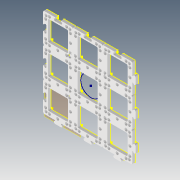
# Autodesk Inventor part: 30_XYTabel_Aliexpress_basplateadapter
Saved by Autodesk Inventor 2022 (Build 260153000, 153)
## iProperties
Created: 2021-11-18
Part Number: 30_XYTabel_Aliexpress_basplateadapter
Material: Generic
Document SubType Name: Modeling
Designer: diederichbenedict
Density: 1 g/cm^3
Appearance: Default
Author: diederichbenedict
Autodesk Inventor part; units mm, degrees
(part 1 of 2)
ref_plane "YZ Plane" through (0, 0, 0) normal (1, 0, 0) x (0, 1, 0)
ref_plane "XZ Plane" through (0, 0, 0) normal (0, 1, 0) x (-1, 0, 0)
ref_plane "XY Plane" through (0, 0, 0) normal (0, 0, 1) x (1, 0, 0)
ref_plane "Work Plane2" through (-50, -50, 0) normal (0, 0, 1) x (1, 0, 0)
sketch "Sketch3" plane through (-50, -50, 0) normal (0, 0, 1) x (1, 0, 0)
  circle A0 centre (5.794757, 15.405243) radius 2.5
  circle A1 centre (-15.605243, -5.794757) radius 2.5
  line L0 (-20.085611, 39.076178) -> (-20.085611, 40.205243)
  line L1 (-20.085611, 40.205243) -> (-38.205243, 40.205243)
  arc A2 (-38.205243, 40.205243) -> (-40.205243, 38.205243) centre (-38.205243, 38.205243) ccw
  line L2 (-40.205243, 20.295345) -> (-40.205243, 38.205243)
  line L3 (-40.205243, 20.295345) -> (-39.078298, 20.295345)
  arc A3 (-39.078298, 20.295345) -> (-38.67683, 20.623155) centre (-39.078298, 20.705088) ccw
  arc A4 (-34.539143, 20.205243) -> (-38.67683, 20.623155) centre (-36.629091, 20.205243) ccw
  line L4 (-34.539143, 20.205243) -> (-34.539143, 10.406652)
  arc A5 (-38.646985, 9.864261) -> (-34.539143, 10.406652) centre (-36.602278, 10.205243) ccw
  line L5 (-38.646985, 9.864261) -> (-38.677461, 9.984929)
  arc A6 (-38.677461, 9.984929) -> (-39.076178, 10.324875) centre (-39.082965, 9.913117) ccw
  line L6 (-39.076178, 10.324875) -> (-40.205243, 10.324875)
  line L7 (-40.205243, -7.794757) -> (-40.205243, 10.324875)
  arc A7 (-40.205243, -7.794757) -> (-38.205243, -9.794757) centre (-38.205243, -7.794757) ccw
  line L8 (-38.205243, -9.794757) -> (-20.205243, -9.794757)
  line L9 (-20.205243, -9.794757) -> (-20.205243, -10.845267)
  arc A8 (-20.605243, -11.335165) -> (-20.205243, -10.845267) centre (-20.705243, -10.845267) ccw
  arc A9 (-20.605243, -11.335165) -> (-20.205243, -15.294757) centre (-20.205243, -13.294757) ccw
  line L10 (-20.205243, -15.294757) -> (-10.205243, -15.294757)
  arc A10 (-10.205243, -15.294757) -> (-9.805243, -11.335165) centre (-10.205243, -13.294757) ccw
  arc A11 (-10.205243, -10.845267) -> (-9.805243, -11.335165) centre (-9.705243, -10.845267) ccw
  line L11 (-10.205243, -10.845267) -> (-10.205243, -9.794757)
  line L12 (-10.205243, -9.794757) -> (7.794757, -9.794757)
  arc A12 (7.794757, -9.794757) -> (9.794757, -7.794757) centre (7.794757, -7.794757) ccw
  line L13 (9.794757, 10.205243) -> (9.794757, -7.794757)
  line L14 (9.794757, 10.205243) -> (10.845267, 10.205243)
  arc A13 (11.335165, 9.805243) -> (10.845267, 10.205243) centre (10.845267, 9.705243) ccw
  arc A14 (11.335165, 9.805243) -> (15.294757, 10.205243) centre (13.294757, 10.205243) ccw
  line L15 (15.294757, 10.205243) -> (15.294757, 20.205243)
  arc A15 (15.294757, 20.205243) -> (11.335165, 20.605243) centre (13.294757, 20.205243) ccw
  arc A16 (10.845267, 20.205243) -> (11.335165, 20.605243) centre (10.845267, 20.705243) ccw
  line L16 (10.845267, 20.205243) -> (9.794757, 20.205243)
  line L17 (9.794757, 38.205243) -> (9.794757, 20.205243)
  arc A17 (9.794757, 38.205243) -> (7.794757, 40.205243) centre (7.794757, 38.205243) ccw
  line L18 (7.794757, 40.205243) -> (-10.115141, 40.205243)
  line L19 (-10.115141, 40.205243) -> (-10.115141, 39.078298)
  arc A18 (-10.115141, 39.078298) -> (-9.787332, 38.67683) centre (-9.705399, 39.078298) ccw
  arc A19 (-10.205243, 34.539143) -> (-9.787332, 38.67683) centre (-10.205243, 36.629091) ccw
  line L20 (-10.205243, 34.539143) -> (-20.003834, 34.539143)
  arc A20 (-20.546226, 38.646985) -> (-20.003834, 34.539143) centre (-20.205243, 36.602278) ccw
  line L21 (-20.546226, 38.646985) -> (-20.425557, 38.677461)
  arc A21 (-20.425557, 38.677461) -> (-20.085611, 39.076178) centre (-20.497369, 39.082965) ccw
  line L22 (-0.205243, 32.205243) -> (-30.205243, 32.205243)
  arc A22 (1.794757, 30.205243) -> (-0.205243, 32.205243) centre (-0.205243, 30.205243) ccw
  line L23 (1.794757, 30.205243) -> (1.794757, 0.205243)
  arc A23 (-0.205243, -1.794757) -> (1.794757, 0.205243) centre (-0.205243, 0.205243) ccw
  line L24 (-0.205243, -1.794757) -> (-30.205243, -1.794757)
  arc A24 (-32.205243, 0.205243) -> (-30.205243, -1.794757) centre (-30.205243, 0.205243) ccw
  line L25 (-32.205243, 0.205243) -> (-32.205243, 30.205243)
  arc A25 (-30.205243, 32.205243) -> (-32.205243, 30.205243) centre (-30.205243, 30.205243) ccw
  circle A26 centre (-35.205243, 35.205243) radius 2.425
  circle A27 centre (-29.705243, 36.005243) radius 2.65 construction
  circle A28 centre (-36.005243, 29.705243) radius 2.65 construction
  circle A29 centre (-35.205243, -4.794757) radius 2.425
  circle A30 centre (-29.705243, -5.594757) radius 2.65 construction
  circle A31 centre (-36.005243, 0.705243) radius 2.65 construction
  circle A32 centre (4.794757, 35.205243) radius 2.425
  circle A33 centre (-0.705243, 36.005243) radius 2.65 construction
  circle A34 centre (5.594757, 29.705243) radius 2.65 construction
  circle A35 centre (5.594757, 0.705243) radius 2.65 construction
  circle A36 centre (-0.705243, -5.594757) radius 2.65 construction
  circle A37 centre (4.794757, -4.794757) radius 2.425
  circle A38 centre (-0.705243, -5.594757) radius 2.6
  circle A39 centre (-29.705243, -5.594757) radius 2.6
  circle A40 centre (-36.005243, 0.705243) radius 2.6
  circle A41 centre (-36.005243, 29.705243) radius 2.6
  circle A42 centre (-29.705243, 36.005243) radius 2.6
  circle A43 centre (-0.705243, 36.005243) radius 2.6
  circle A44 centre (5.594757, 29.705243) radius 2.6
  circle A45 centre (5.594757, 0.705243) radius 2.6
  point P0 (50, 50)
  dimension "d23" = 0.05
  dimension "d24" = 0.05
  dimension "d25" = 0.05
  dimension "d26" = 0.05
  dimension "d27" = 0.05
  dimension "d28" = 0.05
  dimension "d29" = 0.05
  dimension "d30" = 0.05
  constraints: 8 centre point
  measures "d23" radial gap between concentric circles of A36 A38
  measures "d24" radial gap between concentric circles of A30 A39
  measures "d25" radial gap between concentric circles of A31 A40
  measures "d26" radial gap between concentric circles of A28 A41
  measures "d27" radial gap between concentric circles of A27 A42
  measures "d28" radial gap between concentric circles of A33 A43
  measures "d29" radial gap between concentric circles of A34 A44
  measures "d30" radial gap between concentric circles of A35 A45
extrude "Extrusion2" add sketch "Sketch3" along normal blind 5
pattern_linear "Rectangular Pattern1" count 3 spacing 50 along (1, 0, 0) count 3 spacing 50 along (0, 1, 0) of "Extrusion2"
sketch "Sketch4" plane through (-50, -50, 5) normal (0, 0, 1) x (1, 0, 0)
  line L0 (-10.115141, 40.205243) -> (-10.115141, 39.078298)
  arc A0 (-10.115141, 39.078298) -> (-9.787332, 38.67683) centre (-9.705399, 39.078298) ccw
  arc A1 (-10.205243, 34.539143) -> (-9.787332, 38.67683) centre (-10.205243, 36.629091) ccw
  line L1 (-10.205243, 34.539143) -> (-20.003834, 34.539143)
  arc A2 (-21.642091, 38.096455) -> (-20.003834, 34.539143) centre (-20.205243, 36.602278) ccw
  arc A3 (-21.642091, 38.096455) -> (-20.205243, 34.705243) centre (-20.205243, 36.705243) ccw
  line L2 (-20.205243, 34.705243) -> (-10.205243, 34.705243)
  arc A4 (-10.205243, 34.705243) -> (-9.805243, 38.664835) centre (-10.205243, 36.705243) ccw
  arc A5 (-10.205243, 39.154733) -> (-9.805243, 38.664835) centre (-9.705243, 39.154733) ccw
  line L3 (-10.205243, 39.154733) -> (-10.205243, 40.205243)
  line L4 (-10.205243, 40.205243) -> (-10.115141, 40.205243)
  arc A6 (7.794757, 40.205243) -> (9.794757, 42.205243) centre (7.794757, 42.205243) ccw
  arc A7 (9.794757, 42.205243) -> (11.794757, 40.205243) centre (11.794757, 42.205243) ccw
  arc A8 (11.794757, 40.205243) -> (9.794757, 38.205243) centre (11.794757, 38.205243) ccw
  arc A9 (9.794757, 38.205243) -> (7.794757, 40.205243) centre (7.794757, 38.205243) ccw
  line L5 (9.794757, 20.295345) -> (10.921702, 20.295345)
  arc A10 (10.921702, 20.295345) -> (11.32317, 20.623155) centre (10.921702, 20.705088) ccw
  arc A11 (15.460857, 20.205243) -> (11.32317, 20.623155) centre (13.370909, 20.205243) ccw
  line L6 (15.460857, 20.205243) -> (15.460857, 10.406652)
  arc A12 (11.903545, 8.768396) -> (15.460857, 10.406652) centre (13.397722, 10.205243) ccw
  arc A13 (11.903545, 8.768396) -> (15.294757, 10.205243) centre (13.294757, 10.205243) ccw
  line L7 (15.294757, 10.205243) -> (15.294757, 20.205243)
  arc A14 (15.294757, 20.205243) -> (11.335165, 20.605243) centre (13.294757, 20.205243) ccw
  arc A15 (10.845267, 20.205243) -> (11.335165, 20.605243) centre (10.845267, 20.705243) ccw
  line L8 (10.845267, 20.205243) -> (9.794757, 20.205243)
  line L9 (9.794757, 20.205243) -> (9.794757, 20.295345)
  line L10 (39.884859, 90.205243) -> (39.884859, 89.078298)
  arc A16 (39.884859, 89.078298) -> (40.212668, 88.67683) centre (40.294601, 89.078298) ccw
  arc A17 (39.794757, 84.539143) -> (40.212668, 88.67683) centre (39.794757, 86.629091) ccw
  line L11 (39.794757, 84.539143) -> (29.996166, 84.539143)
  arc A18 (28.357909, 88.096455) -> (29.996166, 84.539143) centre (29.794757, 86.602278) ccw
  arc A19 (28.357909, 88.096455) -> (29.794757, 84.705243) centre (29.794757, 86.705243) ccw
  line L12 (29.794757, 84.705243) -> (39.794757, 84.705243)
  arc A20 (39.794757, 84.705243) -> (40.194757, 88.664835) centre (39.794757, 86.705243) ccw
  arc A21 (39.794757, 89.154733) -> (40.194757, 88.664835) centre (40.294757, 89.154733) ccw
  line L13 (39.794757, 89.154733) -> (39.794757, 90.205243)
  line L14 (39.794757, 90.205243) -> (39.884859, 90.205243)
  arc A22 (11.903545, 108.768396) -> (15.294757, 110.205243) centre (13.294757, 110.205243) ccw
  line L15 (15.294757, 110.205243) -> (15.294757, 120.205243)
  arc A23 (15.294757, 120.205243) -> (11.335165, 120.605243) centre (13.294757, 120.205243) ccw
  arc A24 (10.845267, 120.205243) -> (11.335165, 120.605243) centre (10.845267, 120.705243) ccw
  line L16 (10.845267, 120.205243) -> (9.794757, 120.205243)
  line L17 (9.794757, 120.205243) -> (9.794757, 120.295345)
  line L18 (9.794757, 120.295345) -> (10.921702, 120.295345)
  arc A25 (10.921702, 120.295345) -> (11.32317, 120.623155) centre (10.921702, 120.705088) ccw
  arc A26 (15.460857, 120.205243) -> (11.32317, 120.623155) centre (13.370909, 120.205243) ccw
  line L19 (15.460857, 120.205243) -> (15.460857, 110.406652)
  arc A27 (11.903545, 108.768396) -> (15.460857, 110.406652) centre (13.397722, 110.205243) ccw
  arc A28 (9.794757, 92.205243) -> (11.794757, 90.205243) centre (11.794757, 92.205243) ccw
  arc A29 (11.794757, 90.205243) -> (9.794757, 88.205243) centre (11.794757, 88.205243) ccw
  arc A30 (9.794757, 88.205243) -> (7.794757, 90.205243) centre (7.794757, 88.205243) ccw
  arc A31 (7.794757, 90.205243) -> (9.794757, 92.205243) centre (7.794757, 92.205243) ccw
  line L20 (51.794757, 130.205243) -> (51.794757, 100.205243)
  arc A32 (49.794757, 98.205243) -> (51.794757, 100.205243) centre (49.794757, 100.205243) ccw
  line L21 (49.794757, 98.205243) -> (19.794757, 98.205243)
  arc A33 (17.794757, 100.205243) -> (19.794757, 98.205243) centre (19.794757, 100.205243) ccw
  line L22 (17.794757, 100.205243) -> (17.794757, 130.205243)
  arc A34 (19.794757, 132.205243) -> (17.794757, 130.205243) centre (19.794757, 130.205243) ccw
  line L23 (19.794757, 132.205243) -> (49.794757, 132.205243)
  arc A35 (51.794757, 130.205243) -> (49.794757, 132.205243) centre (49.794757, 130.205243) ccw
  circle A36 centre (55.594757, 129.705243) radius 2.6
  circle A37 centre (20.294757, 136.005243) radius 2.6
  circle A38 centre (13.994757, 100.705243) radius 2.6
  circle A39 centre (55.794757, 115.405243) radius 2.5
  circle A40 centre (34.394757, 94.205243) radius 2.5
  circle A41 centre (14.794757, 135.205243) radius 2.425
  circle A42 centre (14.794757, 95.205243) radius 2.425
  circle A43 centre (54.794757, 135.205243) radius 2.425
  circle A44 centre (54.794757, 95.205243) radius 2.425
  circle A45 centre (49.294757, 94.405243) radius 2.6
  circle A46 centre (20.294757, 94.405243) radius 2.6
  circle A47 centre (13.994757, 129.705243) radius 2.6
  circle A48 centre (49.294757, 136.005243) radius 2.6
  circle A49 centre (55.594757, 100.705243) radius 2.6
  line L24 (39.884859, 40.205243) -> (39.884859, 39.078298)
  arc A50 (39.884859, 39.078298) -> (40.212668, 38.67683) centre (40.294601, 39.078298) ccw
  arc A51 (39.794757, 34.539143) -> (40.212668, 38.67683) centre (39.794757, 36.629091) ccw
  line L25 (39.794757, 34.539143) -> (29.996166, 34.539143)
  arc A52 (28.357909, 38.096455) -> (29.996166, 34.539143) centre (29.794757, 36.602278) ccw
  arc A53 (28.357909, 38.096455) -> (29.794757, 34.705243) centre (29.794757, 36.705243) ccw
  line L26 (29.794757, 34.705243) -> (39.794757, 34.705243)
  arc A54 (39.794757, 34.705243) -> (40.194757, 38.664835) centre (39.794757, 36.705243) ccw
  arc A55 (39.794757, 39.154733) -> (40.194757, 38.664835) centre (40.294757, 39.154733) ccw
  line L27 (39.794757, 39.154733) -> (39.794757, 40.205243)
  line L28 (39.794757, 40.205243) -> (39.884859, 40.205243)
  circle A56 centre (5.594757, 50.705243) radius 2.6
  circle A57 centre (-0.705243, 86.005243) radius 2.6
  circle A58 centre (-36.005243, 79.705243) radius 2.6
  circle A59 centre (-29.705243, 44.405243) radius 2.6
  circle A60 centre (-0.705243, 44.405243) radius 2.6
  circle A61 centre (4.794757, 45.205243) radius 2.425
  circle A62 centre (4.794757, 85.205243) radius 2.425
  circle A63 centre (-35.205243, 45.205243) radius 2.425
  circle A64 centre (-35.205243, 85.205243) radius 2.425
  circle A65 centre (-15.605243, 44.205243) radius 2.5
  circle A66 centre (5.794757, 65.405243) radius 2.5
  circle A67 centre (-36.005243, 50.705243) radius 2.6
  circle A68 centre (-29.705243, 86.005243) radius 2.6
  circle A69 centre (5.594757, 79.705243) radius 2.6
  line L29 (1.794757, 80.205243) -> (1.794757, 50.205243)
  arc A70 (-0.205243, 48.205243) -> (1.794757, 50.205243) centre (-0.205243, 50.205243) ccw
  line L30 (-0.205243, 48.205243) -> (-30.205243, 48.205243)
  arc A71 (-32.205243, 50.205243) -> (-30.205243, 48.205243) centre (-30.205243, 50.205243) ccw
  line L31 (-32.205243, 50.205243) -> (-32.205243, 80.205243)
  arc A72 (-30.205243, 82.205243) -> (-32.205243, 80.205243) centre (-30.205243, 80.205243) ccw
  line L32 (-30.205243, 82.205243) -> (-0.205243, 82.205243)
  arc A73 (1.794757, 80.205243) -> (-0.205243, 82.205243) centre (-0.205243, 80.205243) ccw
  line L33 (51.794757, 80.205243) -> (51.794757, 50.205243)
  arc A74 (49.794757, 48.205243) -> (51.794757, 50.205243) centre (49.794757, 50.205243) ccw
  line L34 (49.794757, 48.205243) -> (19.794757, 48.205243)
  arc A75 (17.794757, 50.205243) -> (19.794757, 48.205243) centre (19.794757, 50.205243) ccw
  line L35 (17.794757, 50.205243) -> (17.794757, 80.205243)
  arc A76 (19.794757, 82.205243) -> (17.794757, 80.205243) centre (19.794757, 80.205243) ccw
  line L36 (19.794757, 82.205243) -> (49.794757, 82.205243)
  arc A77 (51.794757, 80.205243) -> (49.794757, 82.205243) centre (49.794757, 80.205243) ccw
  circle A78 centre (55.594757, 79.705243) radius 2.6
  circle A79 centre (20.294757, 86.005243) radius 2.6
  circle A80 centre (13.994757, 50.705243) radius 2.6
  circle A81 centre (55.794757, 65.405243) radius 2.5
  circle A82 centre (34.394757, 44.205243) radius 2.5
  circle A83 centre (14.794757, 85.205243) radius 2.425
  circle A84 centre (14.794757, 45.205243) radius 2.425
  circle A85 centre (54.794757, 85.205243) radius 2.425
  circle A86 centre (54.794757, 45.205243) radius 2.425
  circle A87 centre (49.294757, 44.405243) radius 2.6
  circle A88 centre (20.294757, 44.405243) radius 2.6
  circle A89 centre (13.994757, 79.705243) radius 2.6
  circle A90 centre (49.294757, 86.005243) radius 2.6
  circle A91 centre (55.594757, 50.705243) radius 2.6
  arc A92 (11.903545, 58.768396) -> (15.294757, 60.205243) centre (13.294757, 60.205243) ccw
  line L37 (15.294757, 60.205243) -> (15.294757, 70.205243)
  arc A93 (15.294757, 70.205243) -> (11.335165, 70.605243) centre (13.294757, 70.205243) ccw
  arc A94 (10.845267, 70.205243) -> (11.335165, 70.605243) centre (10.845267, 70.705243) ccw
  line L38 (10.845267, 70.205243) -> (9.794757, 70.205243)
  line L39 (9.794757, 70.205243) -> (9.794757, 70.295345)
  line L40 (9.794757, 70.295345) -> (10.921702, 70.295345)
  arc A95 (10.921702, 70.295345) -> (11.32317, 70.623155) centre (10.921702, 70.705088) ccw
  arc A96 (15.460857, 70.205243) -> (11.32317, 70.623155) centre (13.370909, 70.205243) ccw
  line L41 (15.460857, 70.205243) -> (15.460857, 60.406652)
  arc A97 (11.903545, 58.768396) -> (15.460857, 60.406652) centre (13.397722, 60.205243) ccw
  arc A98 (61.903545, 8.768396) -> (65.294757, 10.205243) centre (63.294757, 10.205243) ccw
  line L42 (65.294757, 10.205243) -> (65.294757, 20.205243)
  arc A99 (65.294757, 20.205243) -> (61.335165, 20.605243) centre (63.294757, 20.205243) ccw
  arc A100 (60.845267, 20.205243) -> (61.335165, 20.605243) centre (60.845267, 20.705243) ccw
  line L43 (60.845267, 20.205243) -> (59.794757, 20.205243)
  line L44 (59.794757, 20.205243) -> (59.794757, 20.295345)
  line L45 (59.794757, 20.295345) -> (60.921702, 20.295345)
  arc A101 (60.921702, 20.295345) -> (61.32317, 20.623155) centre (60.921702, 20.705088) ccw
  arc A102 (65.460857, 20.205243) -> (61.32317, 20.623155) centre (63.370909, 20.205243) ccw
  line L46 (65.460857, 20.205243) -> (65.460857, 10.406652)
  arc A103 (61.903545, 8.768396) -> (65.460857, 10.406652) centre (63.397722, 10.205243) ccw
  line L47 (101.794757, 30.205243) -> (101.794757, 0.205243)
  arc A104 (99.794757, -1.794757) -> (101.794757, 0.205243) centre (99.794757, 0.205243) ccw
  line L48 (99.794757, -1.794757) -> (69.794757, -1.794757)
  arc A105 (67.794757, 0.205243) -> (69.794757, -1.794757) centre (69.794757, 0.205243) ccw
  line L49 (67.794757, 0.205243) -> (67.794757, 30.205243)
  arc A106 (69.794757, 32.205243) -> (67.794757, 30.205243) centre (69.794757, 30.205243) ccw
  line L50 (69.794757, 32.205243) -> (99.794757, 32.205243)
  arc A107 (101.794757, 30.205243) -> (99.794757, 32.205243) centre (99.794757, 30.205243) ccw
  circle A108 centre (105.594757, 29.705243) radius 2.6
  circle A109 centre (70.294757, 36.005243) radius 2.6
  circle A110 centre (63.994757, 0.705243) radius 2.6
  circle A111 centre (105.794757, 15.405243) radius 2.5
  circle A112 centre (84.394757, -5.794757) radius 2.5
  circle A113 centre (64.794757, 35.205243) radius 2.425
  circle A114 centre (64.794757, -4.794757) radius 2.425
  circle A115 centre (104.794757, 35.205243) radius 2.425
  circle A116 centre (104.794757, -4.794757) radius 2.425
  circle A117 centre (99.294757, -5.594757) radius 2.6
  circle A118 centre (70.294757, -5.594757) radius 2.6
  circle A119 centre (63.994757, 29.705243) radius 2.6
  circle A120 centre (99.294757, 36.005243) radius 2.6
  circle A121 centre (105.594757, 0.705243) radius 2.6
  line L51 (51.794757, 30.205243) -> (51.794757, 0.205243)
  arc A122 (49.794757, -1.794757) -> (51.794757, 0.205243) centre (49.794757, 0.205243) ccw
  line L52 (49.794757, -1.794757) -> (19.794757, -1.794757)
  arc A123 (17.794757, 0.205243) -> (19.794757, -1.794757) centre (19.794757, 0.205243) ccw
  line L53 (17.794757, 0.205243) -> (17.794757, 30.205243)
  arc A124 (19.794757, 32.205243) -> (17.794757, 30.205243) centre (19.794757, 30.205243) ccw
  line L54 (19.794757, 32.205243) -> (49.794757, 32.205243)
  arc A125 (51.794757, 30.205243) -> (49.794757, 32.205243) centre (49.794757, 30.205243) ccw
  circle A126 centre (55.594757, 29.705243) radius 2.6
  circle A127 centre (20.294757, 36.005243) radius 2.6
  circle A128 centre (13.994757, 0.705243) radius 2.6
  circle A129 centre (55.794757, 15.405243) radius 2.5
  circle A130 centre (34.394757, -5.794757) radius 2.5
  circle A131 centre (14.794757, 35.205243) radius 2.425
  circle A132 centre (14.794757, -4.794757) radius 2.425
  circle A133 centre (54.794757, 35.205243) radius 2.425
  circle A134 centre (54.794757, -4.794757) radius 2.425
  circle A135 centre (49.294757, -5.594757) radius 2.6
  circle A136 centre (20.294757, -5.594757) radius 2.6
  circle A137 centre (13.994757, 29.705243) radius 2.6
  circle A138 centre (49.294757, 36.005243) radius 2.6
  circle A139 centre (55.594757, 0.705243) radius 2.6
  circle A140 centre (105.594757, 50.705243) radius 2.6
  circle A141 centre (99.294757, 86.005243) radius 2.6
  circle A142 centre (63.994757, 79.705243) radius 2.6
  circle A143 centre (70.294757, 44.405243) radius 2.6
  circle A144 centre (99.294757, 44.405243) radius 2.6
  circle A145 centre (104.794757, 45.205243) radius 2.425
  circle A146 centre (104.794757, 85.205243) radius 2.425
  circle A147 centre (64.794757, 45.205243) radius 2.425
  circle A148 centre (64.794757, 85.205243) radius 2.425
  circle A149 centre (84.394757, 44.205243) radius 2.5
  circle A150 centre (105.794757, 65.405243) radius 2.5
  circle A151 centre (63.994757, 50.705243) radius 2.6
  circle A152 centre (70.294757, 86.005243) radius 2.6
  circle A153 centre (105.594757, 79.705243) radius 2.6
  line L55 (101.794757, 80.205243) -> (101.794757, 50.205243)
  arc A154 (99.794757, 48.205243) -> (101.794757, 50.205243) centre (99.794757, 50.205243) ccw
  line L56 (99.794757, 48.205243) -> (69.794757, 48.205243)
  arc A155 (67.794757, 50.205243) -> (69.794757, 48.205243) centre (69.794757, 50.205243) ccw
  line L57 (67.794757, 50.205243) -> (67.794757, 80.205243)
  arc A156 (69.794757, 82.205243) -> (67.794757, 80.205243) centre (69.794757, 80.205243) ccw
  line L58 (69.794757, 82.205243) -> (99.794757, 82.205243)
  arc A157 (101.794757, 80.205243) -> (99.794757, 82.205243) centre (99.794757, 80.205243) ccw
  arc A158 (59.794757, 42.205243) -> (61.794757, 40.205243) centre (61.794757, 42.205243) ccw
  arc A159 (61.794757, 40.205243) -> (59.794757, 38.205243) centre (61.794757, 38.205243) ccw
  arc A160 (59.794757, 38.205243) -> (57.794757, 40.205243) centre (57.794757, 38.205243) ccw
  arc A161 (57.794757, 40.205243) -> (59.794757, 42.205243) centre (57.794757, 42.205243) ccw
  arc A162 (61.903545, 58.768396) -> (65.294757, 60.205243) centre (63.294757, 60.205243) ccw
  line L59 (65.294757, 60.205243) -> (65.294757, 70.205243)
  arc A163 (65.294757, 70.205243) -> (61.335165, 70.605243) centre (63.294757, 70.205243) ccw
  arc A164 (60.845267, 70.205243) -> (61.335165, 70.605243) centre (60.845267, 70.705243) ccw
  line L60 (60.845267, 70.205243) -> (59.794757, 70.205243)
  line L61 (59.794757, 70.205243) -> (59.794757, 70.295345)
  line L62 (59.794757, 70.295345) -> (60.921702, 70.295345)
  arc A165 (60.921702, 70.295345) -> (61.32317, 70.623155) centre (60.921702, 70.705088) ccw
  arc A166 (65.460857, 70.205243) -> (61.32317, 70.623155) centre (63.370909, 70.205243) ccw
  line L63 (65.460857, 70.205243) -> (65.460857, 60.406652)
  arc A167 (61.903545, 58.768396) -> (65.460857, 60.406652) centre (63.397722, 60.205243) ccw
  line L64 (89.884859, 40.205243) -> (89.884859, 39.078298)
  arc A168 (89.884859, 39.078298) -> (90.212668, 38.67683) centre (90.294601, 39.078298) ccw
  arc A169 (89.794757, 34.539143) -> (90.212668, 38.67683) centre (89.794757, 36.629091) ccw
  line L65 (89.794757, 34.539143) -> (79.996166, 34.539143)
  arc A170 (78.357909, 38.096455) -> (79.996166, 34.539143) centre (79.794757, 36.602278) ccw
  arc A171 (78.357909, 38.096455) -> (79.794757, 34.705243) centre (79.794757, 36.705243) ccw
  line L66 (79.794757, 34.705243) -> (89.794757, 34.705243)
  arc A172 (89.794757, 34.705243) -> (90.194757, 38.664835) centre (89.794757, 36.705243) ccw
  arc A173 (89.794757, 39.154733) -> (90.194757, 38.664835) centre (90.294757, 39.154733) ccw
  line L67 (89.794757, 39.154733) -> (89.794757, 40.205243)
  line L68 (89.794757, 40.205243) -> (89.884859, 40.205243)
  line L69 (1.794757, 130.205243) -> (1.794757, 100.205243)
  arc A174 (-0.205243, 98.205243) -> (1.794757, 100.205243) centre (-0.205243, 100.205243) ccw
  line L70 (-0.205243, 98.205243) -> (-30.205243, 98.205243)
  arc A175 (-32.205243, 100.205243) -> (-30.205243, 98.205243) centre (-30.205243, 100.205243) ccw
  line L71 (-32.205243, 100.205243) -> (-32.205243, 130.205243)
  arc A176 (-30.205243, 132.205243) -> (-32.205243, 130.205243) centre (-30.205243, 130.205243) ccw
  line L72 (-30.205243, 132.205243) -> (-0.205243, 132.205243)
  arc A177 (1.794757, 130.205243) -> (-0.205243, 132.205243) centre (-0.205243, 130.205243) ccw
  circle A178 centre (5.594757, 129.705243) radius 2.6
  circle A179 centre (-29.705243, 136.005243) radius 2.6
  circle A180 centre (-36.005243, 100.705243) radius 2.6
  circle A181 centre (5.794757, 115.405243) radius 2.5
  circle A182 centre (-15.605243, 94.205243) radius 2.5
  circle A183 centre (-35.205243, 135.205243) radius 2.425
  circle A184 centre (-35.205243, 95.205243) radius 2.425
  circle A185 centre (4.794757, 135.205243) radius 2.425
  circle A186 centre (4.794757, 95.205243) radius 2.425
  circle A187 centre (-0.705243, 94.405243) radius 2.6
  circle A188 centre (-29.705243, 94.405243) radius 2.6
  circle A189 centre (-36.005243, 129.705243) radius 2.6
  circle A190 centre (-0.705243, 136.005243) radius 2.6
  circle A191 centre (5.594757, 100.705243) radius 2.6
  line L73 (-10.115141, 90.205243) -> (-10.115141, 89.078298)
  arc A192 (-10.115141, 89.078298) -> (-9.787332, 88.67683) centre (-9.705399, 89.078298) ccw
  arc A193 (-10.205243, 84.539143) -> (-9.787332, 88.67683) centre (-10.205243, 86.629091) ccw
  line L74 (-10.205243, 84.539143) -> (-20.003834, 84.539143)
  arc A194 (-21.642091, 88.096455) -> (-20.003834, 84.539143) centre (-20.205243, 86.602278) ccw
  arc A195 (-21.642091, 88.096455) -> (-20.205243, 84.705243) centre (-20.205243, 86.705243) ccw
  line L75 (-20.205243, 84.705243) -> (-10.205243, 84.705243)
  arc A196 (-10.205243, 84.705243) -> (-9.805243, 88.664835) centre (-10.205243, 86.705243) ccw
  arc A197 (-10.205243, 89.154733) -> (-9.805243, 88.664835) centre (-9.705243, 89.154733) ccw
  line L76 (-10.205243, 89.154733) -> (-10.205243, 90.205243)
  line L77 (-10.205243, 90.205243) -> (-10.115141, 90.205243)
  circle A198 centre (105.594757, 100.705243) radius 2.6
  circle A199 centre (99.294757, 136.005243) radius 2.6
  circle A200 centre (63.994757, 129.705243) radius 2.6
  circle A201 centre (70.294757, 94.405243) radius 2.6
  circle A202 centre (99.294757, 94.405243) radius 2.6
  circle A203 centre (104.794757, 95.205243) radius 2.425
  circle A204 centre (104.794757, 135.205243) radius 2.425
  circle A205 centre (64.794757, 95.205243) radius 2.425
  circle A206 centre (64.794757, 135.205243) radius 2.425
  circle A207 centre (84.394757, 94.205243) radius 2.5
  circle A208 centre (105.794757, 115.405243) radius 2.5
  circle A209 centre (63.994757, 100.705243) radius 2.6
  circle A210 centre (70.294757, 136.005243) radius 2.6
  circle A211 centre (105.594757, 129.705243) radius 2.6
  line L78 (101.794757, 130.205243) -> (101.794757, 100.205243)
  arc A212 (99.794757, 98.205243) -> (101.794757, 100.205243) centre (99.794757, 100.205243) ccw
  line L79 (99.794757, 98.205243) -> (69.794757, 98.205243)
  arc A213 (67.794757, 100.205243) -> (69.794757, 98.205243) centre (69.794757, 100.205243) ccw
  line L80 (67.794757, 100.205243) -> (67.794757, 130.205243)
  arc A214 (69.794757, 132.205243) -> (67.794757, 130.205243) centre (69.794757, 130.205243) ccw
  line L81 (69.794757, 132.205243) -> (99.794757, 132.205243)
  arc A215 (101.794757, 130.205243) -> (99.794757, 132.205243) centre (99.794757, 130.205243) ccw
  arc A216 (59.794757, 92.205243) -> (61.794757, 90.205243) centre (61.794757, 92.205243) ccw
  arc A217 (61.794757, 90.205243) -> (59.794757, 88.205243) centre (61.794757, 88.205243) ccw
  arc A218 (59.794757, 88.205243) -> (57.794757, 90.205243) centre (57.794757, 88.205243) ccw
  arc A219 (57.794757, 90.205243) -> (59.794757, 92.205243) centre (57.794757, 92.205243) ccw
  arc A220 (61.903545, 108.768396) -> (65.294757, 110.205243) centre (63.294757, 110.205243) ccw
  line L82 (65.294757, 110.205243) -> (65.294757, 120.205243)
  arc A221 (65.294757, 120.205243) -> (61.335165, 120.605243) centre (63.294757, 120.205243) ccw
  arc A222 (60.845267, 120.205243) -> (61.335165, 120.605243) centre (60.845267, 120.705243) ccw
  line L83 (60.845267, 120.205243) -> (59.794757, 120.205243)
  line L84 (59.794757, 120.205243) -> (59.794757, 120.295345)
  line L85 (59.794757, 120.295345) -> (60.921702, 120.295345)
  arc A223 (60.921702, 120.295345) -> (61.32317, 120.623155) centre (60.921702, 120.705088) ccw
  arc A224 (65.460857, 120.205243) -> (61.32317, 120.623155) centre (63.370909, 120.205243) ccw
  line L86 (65.460857, 120.205243) -> (65.460857, 110.406652)
  arc A225 (61.903545, 108.768396) -> (65.460857, 110.406652) centre (63.397722, 110.205243) ccw
  line L87 (89.884859, 90.205243) -> (89.884859, 89.078298)
  arc A226 (89.884859, 89.078298) -> (90.212668, 88.67683) centre (90.294601, 89.078298) ccw
  arc A227 (89.794757, 84.539143) -> (90.212668, 88.67683) centre (89.794757, 86.629091) ccw
  line L88 (89.794757, 84.539143) -> (79.996166, 84.539143)
  arc A228 (78.357909, 88.096455) -> (79.996166, 84.539143) centre (79.794757, 86.602278) ccw
  arc A229 (78.357909, 88.096455) -> (79.794757, 84.705243) centre (79.794757, 86.705243) ccw
  line L89 (79.794757, 84.705243) -> (89.794757, 84.705243)
  arc A230 (89.794757, 84.705243) -> (90.194757, 88.664835) centre (89.794757, 86.705243) ccw
  arc A231 (89.794757, 89.154733) -> (90.194757, 88.664835) centre (90.294757, 89.154733) ccw
  line L90 (89.794757, 89.154733) -> (89.794757, 90.205243)
  line L91 (89.794757, 90.205243) -> (89.884859, 90.205243)
  line L92 (1.794757, 30.205243) -> (1.794757, 0.205243)
  arc A232 (-0.205243, -1.794757) -> (1.794757, 0.205243) centre (-0.205243, 0.205243) ccw
  line L93 (-0.205243, -1.794757) -> (-30.205243, -1.794757)
  arc A233 (-32.205243, 0.205243) -> (-30.205243, -1.794757) centre (-30.205243, 0.205243) ccw
  line L94 (-32.205243, 0.205243) -> (-32.205243, 30.205243)
  arc A234 (-30.205243, 32.205243) -> (-32.205243, 30.205243) centre (-30.205243, 30.205243) ccw
  line L95 (-30.205243, 32.205243) -> (-0.205243, 32.205243)
  arc A235 (1.794757, 30.205243) -> (-0.205243, 32.205243) centre (-0.205243, 30.205243) ccw
  circle A236 centre (5.594757, 29.705243) radius 2.6
  circle A237 centre (-29.705243, 36.005243) radius 2.6
  circle A238 centre (-36.005243, 0.705243) radius 2.6
  circle A239 centre (5.794757, 15.405243) radius 2.5
  circle A240 centre (-15.605243, -5.794757) radius 2.5
  circle A241 centre (-35.205243, 35.205243) radius 2.425
  circle A242 centre (-35.205243, -4.794757) radius 2.425
  circle A243 centre (4.794757, 35.205243) radius 2.425
  circle A244 centre (4.794757, -4.794757) radius 2.425
  circle A245 centre (-0.705243, -5.594757) radius 2.6
  circle A246 centre (-29.705243, -5.594757) radius 2.6
  circle A247 centre (-36.005243, 29.705243) radius 2.6
  circle A248 centre (-0.705243, 36.005243) radius 2.6
  circle A249 centre (5.594757, 0.705243) radius 2.6
  arc A250 (9.794757, -7.794757) -> (11.794757, -9.794757) centre (11.794757, -7.794757) ccw
  line L96 (11.794757, -9.794757) -> (29.794757, -9.794757)
  line L97 (29.794757, -9.794757) -> (29.794757, -10.845267)
  arc A251 (29.394757, -11.335165) -> (29.794757, -10.845267) centre (29.294757, -10.845267) ccw
  arc A252 (29.394757, -11.335165) -> (29.794757, -15.294757) centre (29.794757, -13.294757) ccw
  line L98 (29.794757, -15.294757) -> (39.794757, -15.294757)
  arc A253 (39.794757, -15.294757) -> (40.194757, -11.335165) centre (39.794757, -13.294757) ccw
  arc A254 (39.794757, -10.845267) -> (40.194757, -11.335165) centre (40.294757, -10.845267) ccw
  line L99 (39.794757, -10.845267) -> (39.794757, -9.794757)
  line L100 (39.794757, -9.794757) -> (57.794757, -9.794757)
  arc A255 (57.794757, -9.794757) -> (59.794757, -7.794757) centre (57.794757, -7.794757) ccw
  arc A256 (59.794757, -7.794757) -> (61.794757, -9.794757) centre (61.794757, -7.794757) ccw
  line L101 (61.794757, -9.794757) -> (79.794757, -9.794757)
  line L102 (79.794757, -9.794757) -> (79.794757, -10.845267)
  arc A257 (79.394757, -11.335165) -> (79.794757, -10.845267) centre (79.294757, -10.845267) ccw
  arc A258 (79.394757, -11.335165) -> (79.794757, -15.294757) centre (79.794757, -13.294757) ccw
  line L103 (79.794757, -15.294757) -> (89.794757, -15.294757)
  arc A259 (89.794757, -15.294757) -> (90.194757, -11.335165) centre (89.794757, -13.294757) ccw
  arc A260 (89.794757, -10.845267) -> (90.194757, -11.335165) centre (90.294757, -10.845267) ccw
  line L104 (89.794757, -10.845267) -> (89.794757, -9.794757)
  line L105 (89.794757, -9.794757) -> (107.794757, -9.794757)
  arc A261 (107.794757, -9.794757) -> (109.794757, -7.794757) centre (107.794757, -7.794757) ccw
  line L106 (109.794757, -7.794757) -> (109.794757, 10.205243)
  line L107 (109.794757, 10.205243) -> (110.845267, 10.205243)
  arc A262 (111.335165, 9.805243) -> (110.845267, 10.205243) centre (110.845267, 9.705243) ccw
  arc A263 (111.335165, 9.805243) -> (115.294757, 10.205243) centre (113.294757, 10.205243) ccw
  line L108 (115.294757, 10.205243) -> (115.294757, 20.205243)
  arc A264 (115.294757, 20.205243) -> (111.335165, 20.605243) centre (113.294757, 20.205243) ccw
  arc A265 (110.845267, 20.205243) -> (111.335165, 20.605243) centre (110.845267, 20.705243) ccw
  line L109 (110.845267, 20.205243) -> (109.794757, 20.205243)
  line L110 (109.794757, 20.205243) -> (109.794757, 38.205243)
  arc A266 (109.794757, 38.205243) -> (107.794757, 40.205243) centre (107.794757, 38.205243) ccw
  arc A267 (107.794757, 40.205243) -> (109.794757, 42.205243) centre (107.794757, 42.205243) ccw
  line L111 (109.794757, 42.205243) -> (109.794757, 60.205243)
  line L112 (109.794757, 60.205243) -> (110.845267, 60.205243)
  arc A268 (111.335165, 59.805243) -> (110.845267, 60.205243) centre (110.845267, 59.705243) ccw
  arc A269 (111.335165, 59.805243) -> (115.294757, 60.205243) centre (113.294757, 60.205243) ccw
  line L113 (115.294757, 60.205243) -> (115.294757, 70.205243)
  arc A270 (115.294757, 70.205243) -> (111.335165, 70.605243) centre (113.294757, 70.205243) ccw
  arc A271 (110.845267, 70.205243) -> (111.335165, 70.605243) centre (110.845267, 70.705243) ccw
  line L114 (110.845267, 70.205243) -> (109.794757, 70.205243)
  line L115 (109.794757, 70.205243) -> (109.794757, 88.205243)
  arc A272 (109.794757, 88.205243) -> (107.794757, 90.205243) centre (107.794757, 88.205243) ccw
  arc A273 (107.794757, 90.205243) -> (109.794757, 92.205243) centre (107.794757, 92.205243) ccw
  line L116 (109.794757, 92.205243) -> (109.794757, 110.205243)
  line L117 (109.794757, 110.205243) -> (110.845267, 110.205243)
  arc A274 (111.335165, 109.805243) -> (110.845267, 110.205243) centre (110.845267, 109.705243) ccw
  arc A275 (111.335165, 109.805243) -> (115.294757, 110.205243) centre (113.294757, 110.205243) ccw
  line L118 (115.294757, 110.205243) -> (115.294757, 120.205243)
  arc A276 (115.294757, 120.205243) -> (111.335165, 120.605243) centre (113.294757, 120.205243) ccw
  arc A277 (110.845267, 120.205243) -> (111.335165, 120.605243) centre (110.845267, 120.705243) ccw
  line L119 (110.845267, 120.205243) -> (109.794757, 120.205243)
  line L120 (109.794757, 120.205243) -> (109.794757, 138.205243)
  arc A278 (109.794757, 138.205243) -> (107.794757, 140.205243) centre (107.794757, 138.205243) ccw
  line L121 (107.794757, 140.205243) -> (89.884859, 140.205243)
  line L122 (89.884859, 140.205243) -> (89.884859, 139.078298)
  arc A279 (89.884859, 139.078298) -> (90.212668, 138.67683) centre (90.294601, 139.078298) ccw
  arc A280 (89.794757, 134.539143) -> (90.212668, 138.67683) centre (89.794757, 136.629091) ccw
  line L123 (89.794757, 134.539143) -> (79.996166, 134.539143)
  arc A281 (79.453774, 138.646985) -> (79.996166, 134.539143) centre (79.794757, 136.602278) ccw
  line L124 (79.453774, 138.646985) -> (79.574443, 138.677461)
  arc A282 (79.574443, 138.677461) -> (79.914389, 139.076178) centre (79.502631, 139.082965) ccw
  line L125 (79.914389, 139.076178) -> (79.914389, 140.205243)
  line L126 (79.914389, 140.205243) -> (61.794757, 140.205243)
  arc A283 (61.794757, 140.205243) -> (59.794757, 138.205243) centre (61.794757, 138.205243) ccw
  arc A284 (59.794757, 138.205243) -> (57.794757, 140.205243) centre (57.794757, 138.205243) ccw
  line L127 (57.794757, 140.205243) -> (39.884859, 140.205243)
  line L128 (39.884859, 140.205243) -> (39.884859, 139.078298)
  arc A285 (39.884859, 139.078298) -> (40.212668, 138.67683) centre (40.294601, 139.078298) ccw
  arc A286 (39.794757, 134.539143) -> (40.212668, 138.67683) centre (39.794757, 136.629091) ccw
  line L129 (39.794757, 134.539143) -> (29.996166, 134.539143)
  arc A287 (29.453774, 138.646985) -> (29.996166, 134.539143) centre (29.794757, 136.602278) ccw
  line L130 (29.453774, 138.646985) -> (29.574443, 138.677461)
  arc A288 (29.574443, 138.677461) -> (29.914389, 139.076178) centre (29.502631, 139.082965) ccw
  line L131 (29.914389, 139.076178) -> (29.914389, 140.205243)
  line L132 (29.914389, 140.205243) -> (11.794757, 140.205243)
  arc A289 (11.794757, 140.205243) -> (9.794757, 138.205243) centre (11.794757, 138.205243) ccw
  arc A290 (9.794757, 138.205243) -> (7.794757, 140.205243) centre (7.794757, 138.205243) ccw
  line L133 (7.794757, 140.205243) -> (-10.115141, 140.205243)
  line L134 (-10.115141, 140.205243) -> (-10.115141, 139.078298)
  arc A291 (-10.115141, 139.078298) -> (-9.787332, 138.67683) centre (-9.705399, 139.078298) ccw
  arc A292 (-10.205243, 134.539143) -> (-9.787332, 138.67683) centre (-10.205243, 136.629091) ccw
  line L135 (-10.205243, 134.539143) -> (-20.003834, 134.539143)
  arc A293 (-20.546226, 138.646985) -> (-20.003834, 134.539143) centre (-20.205243, 136.602278) ccw
  line L136 (-20.546226, 138.646985) -> (-20.425557, 138.677461)
  arc A294 (-20.425557, 138.677461) -> (-20.085611, 139.076178) centre (-20.497369, 139.082965) ccw
  line L137 (-20.085611, 139.076178) -> (-20.085611, 140.205243)
  line L138 (-20.085611, 140.205243) -> (-38.205243, 140.205243)
  arc A295 (-38.205243, 140.205243) -> (-40.205243, 138.205243) centre (-38.205243, 138.205243) ccw
  line L139 (-40.205243, 138.205243) -> (-40.205243, 120.295345)
  line L140 (-40.205243, 120.295345) -> (-39.078298, 120.295345)
  arc A296 (-39.078298, 120.295345) -> (-38.67683, 120.623155) centre (-39.078298, 120.705088) ccw
  arc A297 (-34.539143, 120.205243) -> (-38.67683, 120.623155) centre (-36.629091, 120.205243) ccw
  line L141 (-34.539143, 120.205243) -> (-34.539143, 110.406652)
  arc A298 (-38.646985, 109.864261) -> (-34.539143, 110.406652) centre (-36.602278, 110.205243) ccw
  line L142 (-38.646985, 109.864261) -> (-38.677461, 109.984929)
  arc A299 (-38.677461, 109.984929) -> (-39.076178, 110.324875) centre (-39.082965, 109.913117) ccw
  line L143 (-39.076178, 110.324875) -> (-40.205243, 110.324875)
  line L144 (-40.205243, 110.324875) -> (-40.205243, 92.205243)
  arc A300 (-40.205243, 92.205243) -> (-38.205243, 90.205243) centre (-38.205243, 92.205243) ccw
  arc A301 (-38.205243, 90.205243) -> (-40.205243, 88.205243) centre (-38.205243, 88.205243) ccw
  line L145 (-40.205243, 88.205243) -> (-40.205243, 70.295345)
  line L146 (-40.205243, 70.295345) -> (-39.078298, 70.295345)
  arc A302 (-39.078298, 70.295345) -> (-38.67683, 70.623155) centre (-39.078298, 70.705088) ccw
  arc A303 (-34.539143, 70.205243) -> (-38.67683, 70.623155) centre (-36.629091, 70.205243) ccw
  line L147 (-34.539143, 70.205243) -> (-34.539143, 60.406652)
  arc A304 (-38.646985, 59.864261) -> (-34.539143, 60.406652) centre (-36.602278, 60.205243) ccw
  line L148 (-38.646985, 59.864261) -> (-38.677461, 59.984929)
  arc A305 (-38.677461, 59.984929) -> (-39.076178, 60.324875) centre (-39.082965, 59.913117) ccw
  line L149 (-39.076178, 60.324875) -> (-40.205243, 60.324875)
  line L150 (-40.205243, 60.324875) -> (-40.205243, 42.205243)
  arc A306 (-40.205243, 42.205243) -> (-38.205243, 40.205243) centre (-38.205243, 42.205243) ccw
  arc A307 (-38.205243, 40.205243) -> (-40.205243, 38.205243) centre (-38.205243, 38.205243) ccw
  line L151 (-40.205243, 38.205243) -> (-40.205243, 20.295345)
  line L152 (-40.205243, 20.295345) -> (-39.078298, 20.295345)
  arc A308 (-39.078298, 20.295345) -> (-38.67683, 20.623155) centre (-39.078298, 20.705088) ccw
  arc A309 (-34.539143, 20.205243) -> (-38.67683, 20.623155) centre (-36.629091, 20.205243) ccw
  line L153 (-34.539143, 20.205243) -> (-34.539143, 10.406652)
  arc A310 (-38.646985, 9.864261) -> (-34.539143, 10.406652) centre (-36.602278, 10.205243) ccw
  line L154 (-38.646985, 9.864261) -> (-38.677461, 9.984929)
  arc A311 (-38.677461, 9.984929) -> (-39.076178, 10.324875) centre (-39.082965, 9.913117) ccw
  line L155 (-39.076178, 10.324875) -> (-40.205243, 10.324875)
  line L156 (-40.205243, 10.324875) -> (-40.205243, -7.794757)
  arc A312 (-40.205243, -7.794757) -> (-38.205243, -9.794757) centre (-38.205243, -7.794757) ccw
  line L157 (-38.205243, -9.794757) -> (-20.205243, -9.794757)
  line L158 (-20.205243, -9.794757) -> (-20.205243, -10.845267)
  arc A313 (-20.605243, -11.335165) -> (-20.205243, -10.845267) centre (-20.705243, -10.845267) ccw
  arc A314 (-20.605243, -11.335165) -> (-20.205243, -15.294757) centre (-20.205243, -13.294757) ccw
  line L159 (-20.205243, -15.294757) -> (-10.205243, -15.294757)
  arc A315 (-10.205243, -15.294757) -> (-9.805243, -11.335165) centre (-10.205243, -13.294757) ccw
  arc A316 (-10.205243, -10.845267) -> (-9.805243, -11.335165) centre (-9.705243, -10.845267) ccw
  line L160 (-10.205243, -10.845267) -> (-10.205243, -9.794757)
  line L161 (-10.205243, -9.794757) -> (7.794757, -9.794757)
  arc A317 (7.794757, -9.794757) -> (9.794757, -7.794757) centre (7.794757, -7.794757) ccw
  point P0 (50, 50)
extrude "Extrusion3" add sketch "Sketch4" against normal blind 5 contours L0 A0 A1 L1 A2 A3 L2 A4 A5 L3 L4 | A6 A7 A8 A9 | L5 A10 A11 L6 A12 A13 L7 A14 A15 L8 L9 | L10 A16 A17 L11 A18 A19 L12 A20 A21 L13 L14 | A22 L15 A23 A24 L16 L17 L18 A25 A26 L19 A27 | A28 A29 A30 A31 | L24 A50 A51 L25 A52 A53 L26 A54 A55 L27 L28 | A92 L37 A93 A94 L38 L39 L40 A95 A96 L41 A97 | A98 L42 A99 A100 L43 L44 L45 A101 A102 L46 A103 | A113 | A158 A159 A160 A161 | A162 L59 A163 A164 L60 L61 L62 A165 A166 L63 A167 | L64 A168 A169 L65 A170 A171 L66 A172 A173 L67 L68 | A186 | L73 A192 A193 L74 A194 A195 L75 A196 A197 L76 L77 | A205 | A216 A217 A218 A219 | A220 L82 A221 A222 L83 L84 L85 A223 A224 L86 A225 | L87 A226 A227 L88 A228 A229 L89 A230 A231 L90 L91 | A243
sketch "Sketch5" plane through (-50, -50, 5) normal (0, 0, 1) x (1, 0, 0)
  circle A0 centre (34.394757, 65.405243) radius 17
  line L0 (4.394757, 95.405243) -> (64.394757, 95.405243) construction
  line L1 (64.394757, 95.405243) -> (64.394757, 35.405243) construction
  line L2 (64.394757, 35.405243) -> (4.394757, 35.405243) construction
  line L3 (4.394757, 35.405243) -> (4.394757, 95.405243) construction
  line L4 (4.394757, 95.405243) -> (64.394757, 35.405243) construction
  line L5 (64.394757, 95.405243) -> (4.394757, 35.405243) construction
  point P0 (50, 50)
  dimension "d39" = 60
  dimension "d40" = 60
  constraints: 12 end point, 2 midpoint, 2 parallel, 1 horizontal, 1 perpendicular
  measures "d39" distance of L1.end L2.end
  measures "d40" distance of L0.end L1.end
hole "Hole2" at (14.394757, -14.594757, 5) at (-45.605243, -14.594757, 5) at (-45.605243, 45.405243, 5) at (14.394757, 45.405243, 5) direction (0, 0, -1) diameter 3 end through all counterbore diameter 6 counterbore depth 3